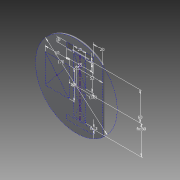
# Autodesk Inventor part: Base Plate
Saved by Autodesk Inventor 2015 (Build 190159000, 159)
## iProperties
Created: 2014-07-27
Part Number: Base Plate
Material: Generic
Document SubType Name: Modeling
Designer: karl
Density: 1 g/cm^3
Appearance: Default
Author: karl
Autodesk Inventor part; units mm, degrees
ref_plane "YZ Plane" through (0, 0, 0) normal (1, 0, 0) x (0, 1, 0)
ref_plane "XZ Plane" through (0, 0, 0) normal (0, 1, 0) x (-1, 0, 0)
ref_plane "XY Plane" through (0, 0, 0) normal (0, 0, 1) x (1, 0, 0)
sketch "Sketch1" plane through (0, 0, 0) normal (0, 1, 0) x (-1, 0, 0)
  circle A0 centre (0, 0) radius 85 construction
  line L0 (-55, 64.8074) -> (-55, -64.8074) construction
  line L1 (-35, 74) -> (23, 74) construction
  line L2 (23, 74) -> (23, 60) construction
  line L3 (23, 60) -> (-35, 60) construction
  line L4 (-35, 60) -> (-35, 74) construction
  line L5 (-35, -60) -> (23, -60) construction
  line L6 (23, -60) -> (23, -74) construction
  line L7 (23, -74) -> (-35, -74) construction
  line L8 (-35, -74) -> (-35, -60) construction
  line L9 (-6, 60) -> (-6, -60)
  line L10 (6.5, 5) -> (-18.5, 5) construction
  line L11 (-18.5, 5) -> (-18.5, 57) construction
  line L12 (-18.5, 57) -> (6.5, 57) construction
  line L13 (6.5, 57) -> (6.5, 5) construction
  line L14 (6.5, 5) -> (-18.5, 57) construction
  line L15 (-18.5, 5) -> (6.5, 57) construction
  line L16 (6.5, -57) -> (-18.5, -57) construction
  line L17 (-18.5, -57) -> (-18.5, -5) construction
  line L18 (-18.5, -5) -> (6.5, -5) construction
  line L19 (6.5, -5) -> (6.5, -57) construction
  line L20 (6.5, -57) -> (-18.5, -5) construction
  line L21 (-18.5, -57) -> (6.5, -5) construction
  line L22 (66.5, -30) -> (16.5, -30) construction
  line L23 (16.5, -30) -> (16.5, 30) construction
  line L24 (16.5, 30) -> (66.5, 30) construction
  line L25 (66.5, 30) -> (66.5, -30) construction
  line L26 (66.5, -30) -> (16.5, 30) construction
  line L27 (16.5, -30) -> (66.5, 30) construction
  point P0 (-6, 31)
  point P1 (-6, -31)
  point P2 (41.5, 0)
  point P3 (-6, 0)
  point P4 (41.5, 0)
  dimension "d0" = 170
  dimension "d1" = 55
  dimension "d2" = 58
  dimension "d3" = 14
  dimension "d4" = 60
  dimension "d5" = 20
  dimension "d6" = 60
  dimension "d7" = 25
  dimension "d8" = 52
  dimension "d9" = 3
  dimension "d10" = 3
  dimension "d11" = 10
  dimension "d12" = 50
  dimension "d13" = 60
  dimension "d14" = 10
  constraints: 56 end point, 10 midpoint, 10 parallel, 5 horizontal, 5 perpendicular, 3 equal length, 2 collinear, 2 point on circle, 2 point on line, 1 centre point, 1 coincident, 1 horizontal alignment, 1 vertical
  measures "d0" diameter of A0
  measures "d1" distance from line of point (0, 0) L0
  measures "d2" distance of L2.end L3.end
  measures "d3" distance of L1.end L2.end
  measures "d4" distance from line of point (0, 0) L3
  measures "d5" distance between parallel lines of L0 L4
  measures "d6" distance from line of point (0, 0) L5
  measures "d7" distance of L11.end L12.end
  measures "d8" distance of L10.end L11.end
  measures "d9" distance between parallel lines of L3 L12
  measures "d10" distance between parallel lines of L5 L16
  measures "d11" distance between parallel lines of L18 L10
  measures "d12" distance of L23.end L24.end
  measures "d13" distance of L22.end L23.end
  measures "d14" distance between parallel lines of L13 L23
sketch "Sketch2" plane through (0, 0, 0) normal (0, 1, 0) x (-1, 0, 0)
  circle A0 centre (0, 0) radius 85 construction
  line L0 (-55, 64.8074) -> (-55, -64.8074) construction
  arc A1 (-55, -64.8074) -> (-55, 64.8074) centre (0, 0) ccw
  line L1 (-55, 64.8074) -> (-55, -64.8074)
  constraints: 2 end point, 2 point on circle, 1 centre point, 1 coincident, 1 collinear, 1 concentric
extrude "Extrusion1" add sketch "Sketch2" along normal blind 3
sketch "Sketch3" plane through (0, 0, 0) normal (0, -1, 0) x (1, 0, 0)
  line L0 (-23, 74) -> (35, 74)
  line L1 (35, 74) -> (35, 60)
  line L2 (35, 60) -> (-23, 60)
  line L3 (-23, 60) -> (-23, 74)
  point P0 (0, 0)
  constraints: 8 end point, 2 parallel, 1 horizontal, 1 perpendicular
extrude "Extrusion2" cut sketch "Sketch3" against normal blind 3
sketch "Sketch4" plane through (0, 0, 0) normal (0, -1, 0) x (1, 0, 0)
  line L0 (-23, 60) -> (-13, 60)
  line L1 (-13, 60) -> (-13, 57)
  line L2 (-13, 57) -> (-23, 57)
  line L3 (-23, 57) -> (-23, 60)
  line L4 (35, 60) -> (25, 60)
  line L5 (25, 60) -> (25, 57)
  line L6 (25, 57) -> (35, 57)
  line L7 (35, 57) -> (35, 60)
  point P0 (0, 0)
  dimension "d19" = 10
  dimension "d20" = 3
  dimension "d21" = 10
  dimension "d22" = 3
  constraints: 16 end point, 4 parallel, 2 horizontal, 2 perpendicular
  measures "d19" distance of L1.end L2.end
  measures "d20" distance of L0.end L1.end
  measures "d21" distance of L6.end L5.end
  measures "d22" distance of L5.end L4.end
extrude "Extrusion3" cut sketch "Sketch4" against normal blind 3
sketch "Sketch5" plane through (0, 0, 0) normal (0, -1, 0) x (1, 0, 0)
  line L0 (18.5, 5) -> (18.5, 57) construction
  line L1 (18.5, 37) -> (21.5, 37)
  line L2 (21.5, 37) -> (21.5, 27)
  line L3 (21.5, 27) -> (18.5, 27)
  line L4 (18.5, 27) -> (18.5, 37)
  line L5 (35, 57) -> (25, 57) projected
  point P0 (0, 0)
  dimension "d25" = 3
  dimension "d26" = 10
  dimension "d27" = 20
  constraints: 8 end point, 2 parallel, 1 horizontal, 1 perpendicular, 1 point on line
  measures "d25" distance of L2.end L3.end
  measures "d26" distance of L1.end L2.end
  measures "d27" distance between parallel lines of L1 L5
extrude "Extrusion4" cut sketch "Sketch5" against normal blind 3
sketch "Sketch6" plane through (0, 0, 0) normal (0, -1, 0) x (1, 0, 0)
  line L0 (-66.5, 30) -> (-66.5, -30) construction
  line L1 (-66.5, 30) -> (-69.5, 30)
  line L2 (-69.5, 30) -> (-69.5, 20)
  line L3 (-69.5, 20) -> (-66.5, 20)
  line L4 (-66.5, 20) -> (-66.5, 30)
  line L5 (-66.5, 5) -> (-69.5, 5)
  line L6 (-69.5, 5) -> (-69.5, -5)
  line L7 (-69.5, -5) -> (-66.5, -5)
  line L8 (-66.5, -5) -> (-66.5, 5)
  line L9 (-66.5, -30) -> (-69.5, -30)
  line L10 (-69.5, -30) -> (-69.5, -20)
  line L11 (-69.5, -20) -> (-66.5, -20)
  line L12 (-66.5, -20) -> (-66.5, -30)
  point P0 (0, 0)
  point P1 (-69.5, 0)
  point P2 (-66.5, 0)
  dimension "d30" = 3
  dimension "d31" = 10
  dimension "d32" = 3
  dimension "d33" = 10
  dimension "d34" = 3
  dimension "d35" = 10
  constraints: 24 end point, 6 parallel, 3 horizontal, 3 perpendicular, 2 midpoint, 1 horizontal alignment, 1 point on line
  measures "d30" distance of L3.end L2.end
  measures "d31" distance of L2.end L1.end
  measures "d32" distance of L7.end L6.end
  measures "d33" distance of L6.end L5.end
  measures "d34" distance of L10.end L11.end
  measures "d35" distance of L9.end L10.end
extrude "Extrusion5" cut sketch "Sketch6" against normal blind 3
sketch "Sketch7" plane through (0, 0, 0) normal (0, -1, 0) x (1, 0, 0)
  line L0 (-16.5, -30) -> (-66.5, 30) construction
  line L1 (-63.5, 26.4) -> (-19.5, 26.4)
  line L2 (-19.5, 26.4) -> (-19.5, -26.4)
  line L3 (-19.5, -26.4) -> (-63.5, -26.4)
  line L4 (-63.5, -26.4) -> (-63.5, 26.4)
  line L5 (-63.5, 26.4) -> (-19.5, -26.4) construction
  line L6 (-19.5, 26.4) -> (-63.5, -26.4) construction
  line L7 (-16.5, -30) -> (-16.5, 30) construction
  circle A0 centre (-19.5, 26.4) radius 1.5
  circle A1 centre (-19.5, -26.4) radius 1.5
  circle A2 centre (-63.5, 26.4) radius 1.5
  circle A3 centre (-63.5, -26.4) radius 1.5
  point P0 (0, 0)
  point P1 (-41.5, 0)
  dimension "d38" = 3
  dimension "d39" = 3
  dimension "d40" = 3
  dimension "d41" = 3
  dimension "d42" = 3
  constraints: 12 end point, 4 centre point, 3 coincident, 3 point on line, 2 midpoint, 2 parallel, 1 horizontal, 1 perpendicular
  measures "d38" distance between parallel lines of L7 L2
  measures "d39" diameter of A0
  measures "d40" diameter of A1
  measures "d41" diameter of A2
  measures "d42" diameter of A3
extrude "Extrusion6" cut sketch "Sketch7" against normal blind 3 contours L4 A2 L1 | L1 A2 L4 | A0 L2 L1 | L1 L2 A0
mirror "Mirror1" about plane through (0, 0, 0) normal (0, 0, 1) of "Extrusion2", "Extrusion3", "Extrusion4", "Extrusion6"
equation "\"d6\" = d4"
equation "\"d10\" = d9"
body "Solid1"
